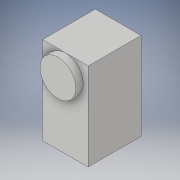
# Autodesk Inventor part: ax_18_replace
Saved by Autodesk Inventor 2018 (Build 220112000, 112)
## iProperties
Created: 2018-10-11
Part Number: ax_18_replace
Material: Generic
Document SubType Name: Modeling
Designer: Abhay
Density: 1 g/cm^3
Appearance: Default
Author: Abhay
Autodesk Inventor part; units mm, degrees
ref_plane "YZ Plane" through (0, 0, 0) normal (1, 0, 0) x (0, 1, 0)
ref_plane "XZ Plane" through (0, 0, 0) normal (0, 1, 0) x (-1, 0, 0)
ref_plane "XY Plane" through (0, 0, 0) normal (0, 0, 1) x (1, 0, 0)
sketch "Sketch1" plane through (0, 0, 0) normal (0, 0, 1) x (1, 0, 0)
  line L0 (0, 0) -> (28, 0)
  line L1 (28, 0) -> (28, -53.6)
  line L2 (28, -53.6) -> (0, -53.6)
  line L3 (0, -53.6) -> (0, 0)
  dimension "d0" = 28
  dimension "d1" = 53.6
  constraints: 8 end point, 2 parallel, 1 horizontal, 1 perpendicular
  measures "d0" distance of L1.end L2.end
  measures "d1" distance of L0.end L1.end
extrude "Extrusion1" add sketch "Sketch1" along normal blind 32.4
sketch "Sketch2" plane through (0, 0, 32.4) normal (0, 0, 1) x (1, 0, 0)
  circle A0 centre (14, -11) radius 11
  dimension "d5" = 22
  constraints: 1 centre point
  measures "d5" diameter of A0
extrude "Extrusion2" add sketch "Sketch2" along normal blind 4.54
sketch "Sketch3" plane through (0, 0, 0) normal (0, 0, -1) x (-1, 0, 0)
  line L0 (0, 0) -> (-28, 0) projected
  line L1 (0, 0) -> (-14, 0)
  line L2 (-14, 0) -> (-14, -11)
  circle A0 centre (-14, -11) radius 5
  dimension "d8" = 14
  dimension "d9" = 11
  dimension "d10" = 10
  constraints: 4 end point, 1 centre point, 1 coincident, 1 midpoint, 1 vertical
  measures "d8" distance of L0.start L1.end
  measures "d9" distance of L1.end L2.end
  measures "d10" diameter of A0
extrude "Extrusion3" add sketch "Sketch3" along normal blind 2.4
sketch "Sketch4" plane through (0, -53.6, 0) normal (0, -1, 0) x (1, 0, 0)
  line L0 (0, 0) -> (28, 0) projected
  line L1 (0, 0) -> (0, 32.4) projected
  line L2 (6.5, 23.7) -> (6.5, 8.7)
  line L3 (6.5, 8.7) -> (21.5, 8.7)
  line L4 (21.5, 8.7) -> (21.5, 23.7)
  circle A0 centre (6.5, 23.7) radius 1.45
  circle A1 centre (6.5, 8.7) radius 1.45
  circle A2 centre (21.5, 8.7) radius 1.45
  circle A3 centre (21.5, 23.7) radius 1.45
  dimension "d17" = 15
  dimension "d18" = 15
  dimension "d19" = 2.9
  dimension "d20" = 2.9
  dimension "d21" = 2.9
  dimension "d22" = 2.9
  constraints: 6 end point, 4 centre point, 4 coincident, 2 perpendicular
  measures "d17" distance of L2.start L2.end
  measures "d18" distance of L2.end L3.end
  measures "d19" diameter of A0
  measures "d20" diameter of A1
  measures "d21" diameter of A2
  measures "d22" diameter of A3
extrude "Extrusion4" add sketch "Sketch4" along normal blind 1
body "Solid1"
